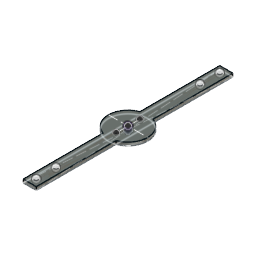
arm (Autodesk Fusion 360 design; units mm, degrees)
Autodesk Fusion 360 part; units mm, degrees
sketch "Sketch1" plane through (0, 0, 0) normal (0, 0, 1) x (1, 0, 0)
  circle A0 centre (0, 0) radius 30
  line L0 (10, 150) -> (-10, 150)
  line L1 (-10, 150) -> (-10, -150)
  line L2 (-10, -150) -> (10, -150)
  line L3 (10, -150) -> (10, 150)
  line L4 (10, 150) -> (-10, -150) construction
  line L5 (-10, 150) -> (10, -150) construction
  dimension "d1" = 60
  dimension "d3" = 20
  dimension "d4" = 300
  constraint coincident A0.centre origin
  constraint horizontal L0
  constraint perpendicular L0 L1
  constraint parallel L0 L2
  constraint parallel L1 L3
  constraint coincident L4 A0.centre
  constraint coincident L5 A0.centre
  measures "d1" diameter of A0
  measures "d3" distance of L0.start L0.end
  measures "d4" distance of L0.end L1.end
extrude "Extrude1" add sketch "Sketch1" along normal blind 5
sketch "Sketch2" plane through (0, 0, 5) normal (0, 0, 1) x (-1, 0, 0)
  line L0 (-10, 150) -> (-10, 28.2843)
  arc A0 (-10, 28.2843) -> (-10, -28.2843) centre (0, 0) ccw
  line L1 (-10, -28.2843) -> (-10, -150)
  line L2 (-10, -150) -> (10, -150)
  line L3 (10, -150) -> (10, -28.2843)
  arc A1 (10, -28.2843) -> (10, 28.2843) centre (0, 0) ccw
  line L4 (10, 28.2843) -> (10, 150)
  line L5 (10, 150) -> (-10, 150)
  line L6 (30, 0) -> (-30, 0) construction
  line L7 (0, -18) -> (0, 18) construction
  point P0 (0, -140)
  point P1 (0, -110)
  point P2 (0, 140)
  point P3 (0, 110)
  point P4 (0, -18)
  point P5 (0, 18)
  dimension "d8" = 30
  dimension "d9" = 10
  dimension "d16" = 36
  constraint coincident A0.centre A1.centre
  constraint midpoint A1 L6.start
  constraint midpoint A0 L6.end
  constraint symmetric P0 L6 P2
  constraint symmetric P1 L6 P3
  constraint coincident P4 L7.start
  constraint coincident P5 L7.end
  constraint vertical L7
  constraint coincident A0.centre L7
  constraint symmetric L6 P4 P5
  measures "d8" distance of P0 P1
  measures "d9" distance of L2 P0
  measures "d16" distance of P4 P5
hole "Hole1" at (0, 0, 5) direction (0, 0, -1) diameter 8.4 end up to surface (5 mm away)
hole "Hole2" at (0, 140, 5) at (0, 110, 5) at (0, -110, 5) at (0, -140, 5) direction (0, 0, -1) diameter 3.2 end up to surface (5 mm away) countersink diameter 5.6 countersink angle 90
hole "Hole3" at (0, 18, 5) at (0, -18, 5) direction (0, 0, -1) diameter 1.8 end up to surface (5 mm away)
